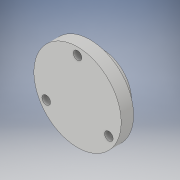
# Autodesk Inventor part: AW7.1 6
Saved by Autodesk Inventor 2018 (Build 220112000, 112)
## iProperties
Created: 2019-01-23
Part Number: AW7.1 6
Material: Generic
Document SubType Name: Modeling
Designer: russd
Density: 1 g/cm^3
Appearance: Default
Author: russd
Autodesk Inventor part; units mm, degrees
ref_plane "YZ Plane" through (0, 0, 0) normal (1, 0, 0) x (0, 1, 0)
ref_plane "XZ Plane" through (0, 0, 0) normal (0, 1, 0) x (-1, 0, 0)
ref_plane "XY Plane" through (0, 0, 0) normal (0, 0, 1) x (1, 0, 0)
sketch "Sketch1" plane through (0, 0, 0) normal (0, 0, 1) x (1, 0, 0)
  circle A0 centre (0, 0) radius 22.225
  circle A1 centre (0, 0) radius 18.415 construction
  circle A2 centre (0, 0) radius 18.415 construction
  circle A3 centre (0, 0) radius 18.415 construction
  circle A4 centre (0, 0) radius 14.7955
  point P0 (0, 18.415)
  point P1 (-15.9479, -9.2075)
  point P2 (15.9479, -9.2075)
  dimension "d1" = 36.83
  dimension "d0" = 44.45
  dimension "d4" = 360
  dimension "d16" = 29.591
  constraints: 3 coincident, 2 centre point, 1 vertical alignment, 18 other
  measures "d0" diameter of A0
  measures "d16" diameter of A4
extrude "Extrusion1" add sketch "Sketch1" along normal blind 6.35 contours A0 | A4
hole "Hole1" at (15.9479, -9.2075, 0) at (0, 18.415, 0) at (-15.9479, -9.2075, 0) direction (0, 0, 1) diameter 4.3688 end through all
extrude "Extrusion2" add sketch "Sketch1" against normal blind 6.35 contours A4
body "Solid1"
